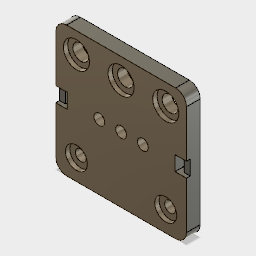
24mm-wheel-2020-gantry (Autodesk Fusion 360 design; units mm, degrees)
Autodesk Fusion 360 part; units mm, degrees
note: some values were not read from the file. Set by a fixed rule: which sketch regions a step uses.
sketch "Sketch1" plane through (0, 0, 0) normal (0, 0, 1) x (1, 0, 0)
  line L0 (30, -30) -> (-30, -30)
  line L1 (-30, -30) -> (-30, 30)
  line L2 (-30, 30) -> (30, 30)
  line L3 (30, 30) -> (30, -30)
  line L4 (30, -30) -> (-30, 30) construction
  line L5 (-30, -30) -> (30, 30) construction
  dimension "d1" = 60
  dimension "d2" = 60
  measures "d1" distance of L0.end L1.end
  measures "d2" distance of L1.end L2.end
extrude "Extrude1" add sketch "Sketch1" along normal blind 6.35
sketch "Sketch2" plane through (0, 0, 6.35) normal (0, 0, 1) x (1, 0, 0)
  line L0 (30, 30) -> (-30, 30)
  line L1 (-30, 30) -> (-30, -30)
  line L2 (-30, -30) -> (30, -30)
  line L3 (30, -30) -> (30, 30)
  line L4 (20.5, -20.5) -> (-20.5, -20.5)
  line L5 (-20.5, -20.5) -> (-20.5, 20.5)
  line L6 (-20.5, 20.5) -> (20.5, 20.5)
  line L7 (20.5, 20.5) -> (20.5, -20.5)
  line L8 (20.5, -20.5) -> (-20.5, 20.5) construction
  line L9 (-20.5, -20.5) -> (20.5, 20.5) construction
  circle A0 centre (-20.5, 20.5) radius 3.575
  circle A1 centre (20.5, 20.5) radius 3.575
  circle A2 centre (20.5, -20.5) radius 2.5
  circle A3 centre (-20.5, -20.5) radius 2.5
  dimension "d5" = 41
  dimension "d6" = 41
  dimension "d7" = 7.15
  dimension "d8" = 7.15
  dimension "d9" = 5
  dimension "d10" = 5
  measures "d5" distance of L4.end L5.end
  measures "d6" distance of L5.end L6.end
  measures "d7" diameter of A0
  measures "d8" diameter of A1
  measures "d9" diameter of A2
  measures "d10" diameter of A3
extrude "Extrude2" cut sketch "Sketch2" against normal through all contours L4 L5 A3 | L4 L5 A3 | L4 L7 A2 | L4 L7 A2 | L5 L6 A0 | L5 L6 A0 | L6 L7 A1 | L6 L7 A1
sketch "Sketch3" plane through (0, 0, 6.35) normal (0, 0, 1) x (1, 0, 0)
  circle A0 centre (-20.5, -20.5) radius 2.5
  circle A1 centre (-20.5, 20.5) radius 3.575
  circle A2 centre (20.5, -20.5) radius 2.5
  circle A3 centre (20.5, 20.5) radius 3.575
  line L0 (30, 30) -> (-30, 30)
  line L1 (-30, 30) -> (-30, -30)
  line L2 (-30, -30) -> (30, -30)
  line L3 (30, -30) -> (30, 30)
  circle A4 centre (-20.5, -20.5) radius 5.05
  circle A5 centre (20.5, -20.5) radius 5.05
  circle A6 centre (20.5, 20.5) radius 5.05
  circle A7 centre (-20.5, 20.5) radius 5.05
  dimension "d12" = 10.1
  dimension "d13" = 10.1
  dimension "d14" = 10.1
  dimension "d15" = 10.1
  measures "d12" diameter of A4
  measures "d13" diameter of A5
  measures "d14" diameter of A6
  measures "d15" diameter of A7
extrude "Extrude3" cut sketch "Sketch3" against normal blind 2 contours A4 | A5 | A6 | A7
fillet "Fillet1" radius 5 2 edges at (30, -30, 3.175) (30, 30, 3.175)
fillet "Fillet2" radius 5 2 edges at (-30, 30, 3.175) (-30, -30, 3.175)
sketch "Sketch4" plane through (0, 0, 6.35) normal (0, 0, 1) x (1, 0, 0)
  arc A0 (-30, -25) -> (-25, -30) centre (-25, -25) ccw
  line L0 (-25, -30) -> (25, -30)
  arc A1 (25, -30) -> (30, -25) centre (25, -25) ccw
  line L1 (30, -25) -> (30, 25)
  arc A2 (30, 25) -> (25, 30) centre (25, 25) ccw
  line L2 (25, 30) -> (-25, 30)
  arc A3 (-25, 30) -> (-30, 25) centre (-25, 25) ccw
  line L3 (-30, 25) -> (-30, -25)
  circle A4 centre (20.5, 20.5) radius 5.05
  circle A5 centre (20.5, -20.5) radius 5.05
  circle A6 centre (-20.5, 20.5) radius 5.05
  circle A7 centre (-20.5, -20.5) radius 5.05
  circle A8 centre (0, 0) radius 2.5
  circle A9 centre (10, 0) radius 2.5
  circle A10 centre (-10, 0) radius 2.5
  line L4 (-25.75, -3.375) -> (-28.25, -3.375)
  line L5 (-28.25, -3.375) -> (-28.25, 3.375)
  line L6 (-28.25, 3.375) -> (-25.75, 3.375)
  line L7 (-25.75, 3.375) -> (-25.75, -3.375)
  line L8 (-25.75, -3.375) -> (-28.25, 3.375) construction
  line L9 (-28.25, -3.375) -> (-25.75, 3.375) construction
  line L10 (28.25, -3.375) -> (25.75, -3.375)
  line L11 (25.75, -3.375) -> (25.75, 3.375)
  line L12 (25.75, 3.375) -> (28.25, 3.375)
  line L13 (28.25, 3.375) -> (28.25, -3.375)
  line L14 (28.25, -3.375) -> (25.75, 3.375) construction
  line L15 (25.75, -3.375) -> (28.25, 3.375) construction
  point P0 (-27, 0)
  point P1 (27, 0)
  dimension "d20" = 5
  dimension "d21" = 5
  dimension "d22" = 5
  dimension "d23" = 6.75
  dimension "d24" = 2.5
  dimension "d25" = 6.75
  dimension "d26" = 2.5
  measures "d20" diameter of A8
  measures "d21" diameter of A9
  measures "d22" diameter of A10
  measures "d23" distance of L4.end L5.end
  measures "d24" distance of L5.end L6.end
  measures "d25" distance of L10.end L11.end
  measures "d26" distance of L11.end L12.end
extrude "Extrude4" cut sketch "Sketch4" against normal through all contours A8 | A9 | A10 | L4 L5 L6 L7 | L10 L11 L12 L13
sketch "Sketch5" plane through (0, 0, 6.35) normal (0, 0, 1) x (1, 0, 0)
  circle A0 centre (0, 0) radius 2.5
  circle A1 centre (-10, 0) radius 2.5
  circle A2 centre (10, 0) radius 2.5
  line L0 (-25.75, 3.375) -> (-25.75, -3.375)
  line L1 (-25.75, -3.375) -> (-28.25, -3.375)
  line L2 (-28.25, -3.375) -> (-28.25, 3.375)
  line L3 (-28.25, 3.375) -> (-25.75, 3.375)
  line L4 (28.25, 3.375) -> (28.25, -3.375)
  line L5 (28.25, -3.375) -> (25.75, -3.375)
  line L6 (25.75, -3.375) -> (25.75, 3.375)
  line L7 (25.75, 3.375) -> (28.25, 3.375)
  arc A3 (-30, -25) -> (-25, -30) centre (-25, -25) ccw
  line L8 (-25, -30) -> (25, -30)
  arc A4 (25, -30) -> (30, -25) centre (25, -25) ccw
  line L9 (30, -25) -> (30, 25)
  arc A5 (30, 25) -> (25, 30) centre (25, 25) ccw
  line L10 (25, 30) -> (-25, 30)
  arc A6 (-25, 30) -> (-30, 25) centre (-25, 25) ccw
  line L11 (-30, 25) -> (-30, -25)
  circle A7 centre (20.5, 20.5) radius 5.05
  circle A8 centre (20.5, -20.5) radius 5.05
  circle A9 centre (-20.5, 20.5) radius 5.05
  circle A10 centre (-20.5, -20.5) radius 5.05
  circle A11 centre (-20.5, 20.5) radius 6
  circle A12 centre (20.5, 20.5) radius 6
  dimension "d28" = 12
  dimension "d29" = 12
  measures "d28" diameter of A11
  measures "d29" diameter of A12
extrude "Extrude5" cut sketch "Sketch5" against normal blind 2 contours A11 | A12
sketch "Sketch6" plane through (0, 0, 6.35) normal (0, 0, 1) x (1, 0, 0)
  circle A0 centre (-20.5, 20.5) radius 6
  circle A1 centre (20.5, 20.5) radius 6
  circle A2 centre (0, 0) radius 2.5
  circle A3 centre (-10, 0) radius 2.5
  circle A4 centre (10, 0) radius 2.5
  line L0 (-25.75, 3.375) -> (-25.75, -3.375)
  line L1 (-25.75, -3.375) -> (-28.25, -3.375)
  line L2 (-28.25, -3.375) -> (-28.25, 3.375)
  line L3 (-28.25, 3.375) -> (-25.75, 3.375)
  line L4 (28.25, 3.375) -> (28.25, -3.375)
  line L5 (28.25, -3.375) -> (25.75, -3.375)
  line L6 (25.75, -3.375) -> (25.75, 3.375)
  line L7 (25.75, 3.375) -> (28.25, 3.375)
  arc A5 (-30, -25) -> (-25, -30) centre (-25, -25) ccw
  line L8 (-25, -30) -> (25, -30)
  arc A6 (25, -30) -> (30, -25) centre (25, -25) ccw
  line L9 (30, -25) -> (30, 25)
  arc A7 (30, 25) -> (25, 30) centre (25, 25) ccw
  line L10 (25, 30) -> (-25, 30)
  arc A8 (-25, 30) -> (-30, 25) centre (-25, 25) ccw
  line L11 (-30, 25) -> (-30, -25)
  circle A9 centre (20.5, -20.5) radius 5.05
  circle A10 centre (-20.5, -20.5) radius 5.05
  circle A11 centre (-20.5, 20.5) radius 3.65
  circle A12 centre (20.5, 20.5) radius 3.65
  dimension "d32" = 7.3
  dimension "d33" = 7.3
  measures "d32" diameter of A11
  measures "d33" diameter of A12
extrude "Extrude6" cut sketch "Sketch6" against normal through all contours A11
sketch "Sketch7" plane through (0, 0, 4.35) normal (0, 0, 1) x (1, 0, 0)
  circle A0 centre (20.5, 20.5) radius 6
  circle A1 centre (20.5, 20.5) radius 3.575
  circle A2 centre (20.5, 20.5) radius 3.65
  dimension "d35" = 7.3
  measures "d35" diameter of A2
extrude "Extrude7" cut sketch "Sketch7" against normal through all contours A2
move_face "OffsetFaces1" offset -1 1 faces at (-25.75, 1.125, 4.2333)
move_face "OffsetFaces2" offset 1 1 faces at (28.25, -1.125, 2.1167)
move_face "OffsetFaces3" offset 1 1 faces at (-28.25, 1.125, 2.1167)
move_face "OffsetFaces4" offset -1 1 faces at (25.75, 1.125, 2.1167)
sketch "Sketch9" plane through (0, 0, 6.35) normal (0, 0, 1) x (1, 0, 0)
  circle A0 centre (-20.5, 20.5) radius 6
  circle A1 centre (20.5, 20.5) radius 6
  circle A2 centre (0, 0) radius 2.5
  circle A3 centre (-10, 0) radius 2.5
  circle A4 centre (10, 0) radius 2.5
  line L0 (-24.75, 3.375) -> (-24.75, -3.375)
  line L1 (-24.75, -3.375) -> (-27.25, -3.375)
  line L2 (-27.25, -3.375) -> (-27.25, 3.375)
  line L3 (-27.25, 3.375) -> (-24.75, 3.375)
  line L4 (27.25, 3.375) -> (27.25, -3.375)
  line L5 (27.25, -3.375) -> (24.75, -3.375)
  line L6 (24.75, -3.375) -> (24.75, 3.375)
  line L7 (24.75, 3.375) -> (27.25, 3.375)
  arc A5 (-30, -25) -> (-25, -30) centre (-25, -25) ccw
  line L8 (-25, -30) -> (25, -30)
  arc A6 (25, -30) -> (30, -25) centre (25, -25) ccw
  line L9 (30, -25) -> (30, 25)
  arc A7 (30, 25) -> (25, 30) centre (25, 25) ccw
  line L10 (25, 30) -> (-25, 30)
  arc A8 (-25, 30) -> (-30, 25) centre (-25, 25) ccw
  line L11 (-30, 25) -> (-30, -25)
  circle A9 centre (20.5, -20.5) radius 5.05
  circle A10 centre (-20.5, -20.5) radius 5.05
  line L12 (-27.25, 3.375) -> (-30, 3.375)
  line L13 (-30, 3.375) -> (-30, -3.375)
  line L14 (-30, -3.375) -> (-27.25, -3.375)
  line L15 (-27.25, -3.375) -> (-27.25, 3.375)
  circle A11 centre (-0.0171, 20.5) radius 3.625
  dimension "d48" = 6.75
  dimension "d51" = 7.25
  measures "d48" distance of L12 L14
  measures "d51" diameter of A11
extrude "Extrude9" cut sketch "Sketch9" against normal blind 1.75 contours L2 L11 L12 L13 L14 L15
sketch "Sketch10" plane through (0, 0, 6.35) normal (0, 0, 1) x (1, 0, 0)
  line L0 (-30, -3.375) -> (-30, -25)
  arc A0 (-30, -25) -> (-25, -30) centre (-25, -25) ccw
  line L1 (-25, -30) -> (25, -30)
  arc A1 (25, -30) -> (30, -25) centre (25, -25) ccw
  line L2 (30, -25) -> (30, 25)
  arc A2 (30, 25) -> (25, 30) centre (25, 25) ccw
  line L3 (25, 30) -> (-25, 30)
  arc A3 (-25, 30) -> (-30, 25) centre (-25, 25) ccw
  line L4 (-30, 25) -> (-30, 3.375)
  line L5 (-30, 3.375) -> (-24.75, 3.375)
  line L6 (-24.75, 3.375) -> (-24.75, -3.375)
  line L7 (-24.75, -3.375) -> (-30, -3.375)
  circle A4 centre (-20.5, 20.5) radius 6
  circle A5 centre (20.5, 20.5) radius 6
  circle A6 centre (0, 0) radius 2.5
  circle A7 centre (-10, 0) radius 2.5
  circle A8 centre (10, 0) radius 2.5
  line L8 (27.25, 3.375) -> (27.25, -3.375)
  line L9 (27.25, -3.375) -> (24.75, -3.375)
  line L10 (24.75, -3.375) -> (24.75, 3.375)
  line L11 (24.75, 3.375) -> (27.25, 3.375)
  circle A9 centre (20.5, -20.5) radius 5.05
  circle A10 centre (-20.5, -20.5) radius 5.05
  line L12 (27.25, 3.375) -> (30, 3.375)
  line L13 (30, 3.375) -> (30, -3.375)
  line L14 (30, -3.375) -> (27.25, -3.375)
  line L15 (27.25, -3.375) -> (27.25, 3.375)
  dimension "d45" = 6.75
  measures "d45" distance of L8.start L8.end
extrude "Extrude10" cut sketch "Sketch10" against normal blind 1.75 contours L2 L8 L12 L13 L14 L15
extrude "Extrude11" cut sketch "Sketch9" against normal blind 1.75 contours L2 L11 L12 L13 L14 L15
extrude "Extrude12" cut sketch "Sketch9" against normal through all contours A11
sketch "Sketch11" plane through (0, 0, 6.35) normal (0, 0, 1) x (1, 0, 0)
  circle A0 centre (-0.0171, 20.5) radius 3.625
  line L0 (30, -3.375) -> (24.75, -3.375)
  line L1 (24.75, -3.375) -> (24.75, 3.375)
  line L2 (24.75, 3.375) -> (30, 3.375)
  line L3 (30, 3.375) -> (30, 25)
  arc A1 (30, 25) -> (25, 30) centre (25, 25) ccw
  line L4 (25, 30) -> (-25, 30)
  arc A2 (-25, 30) -> (-30, 25) centre (-25, 25) ccw
  line L5 (-30, 25) -> (-30, 3.375)
  line L6 (-30, 3.375) -> (-24.75, 3.375)
  line L7 (-24.75, 3.375) -> (-24.75, -3.375)
  line L8 (-24.75, -3.375) -> (-30, -3.375)
  line L9 (-30, -3.375) -> (-30, -25)
  arc A3 (-30, -25) -> (-25, -30) centre (-25, -25) ccw
  line L10 (-25, -30) -> (25, -30)
  arc A4 (25, -30) -> (30, -25) centre (25, -25) ccw
  line L11 (30, -25) -> (30, -3.375)
  circle A5 centre (-20.5, -20.5) radius 5.05
  circle A6 centre (20.5, -20.5) radius 5.05
  circle A7 centre (10, 0) radius 2.5
  circle A8 centre (-10, 0) radius 2.5
  circle A9 centre (0, 0) radius 2.5
  circle A10 centre (20.5, 20.5) radius 6
  circle A11 centre (-20.5, 20.5) radius 6
  circle A12 centre (-0.0171, 20.5) radius 6
  dimension "d53" = 12
  measures "d53" diameter of A12
extrude "Extrude13" cut sketch "Sketch11" against normal blind 2 contours A12
sketch "Sketch12" plane through (0, 0, 6.35) normal (0, 0, 1) x (1, 0, 0)
  circle A0 centre (-0.0171, 20.5) radius 6
  line L0 (30, -3.375) -> (24.75, -3.375)
  line L1 (24.75, -3.375) -> (24.75, 3.375)
  line L2 (24.75, 3.375) -> (30, 3.375)
  line L3 (30, 3.375) -> (30, 25)
  arc A1 (30, 25) -> (25, 30) centre (25, 25) ccw
  line L4 (25, 30) -> (-25, 30)
  arc A2 (-25, 30) -> (-30, 25) centre (-25, 25) ccw
  line L5 (-30, 25) -> (-30, 3.375)
  line L6 (-30, 3.375) -> (-24.75, 3.375)
  line L7 (-24.75, 3.375) -> (-24.75, -3.375)
  line L8 (-24.75, -3.375) -> (-30, -3.375)
  line L9 (-30, -3.375) -> (-30, -25)
  arc A3 (-30, -25) -> (-25, -30) centre (-25, -25) ccw
  line L10 (-25, -30) -> (25, -30)
  arc A4 (25, -30) -> (30, -25) centre (25, -25) ccw
  line L11 (30, -25) -> (30, -3.375)
  circle A5 centre (-20.5, -20.5) radius 5.05
  circle A6 centre (20.5, -20.5) radius 5.05
  circle A7 centre (10, 0) radius 2.5
  circle A8 centre (-10, 0) radius 2.5
  circle A9 centre (0, 0) radius 2.5
  circle A10 centre (20.5, 20.5) radius 6
  circle A11 centre (-20.5, 20.5) radius 6
